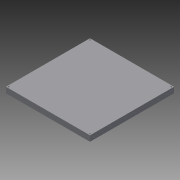
# Autodesk Inventor part: locomotion top
Saved by Autodesk Inventor 2015 (Build 190159000, 159)
## iProperties
Created: 2014-10-23
Part Number: locomotion top
Material: Generic
Document SubType Name: Modeling
Designer: ericd_000
Density: 1 g/cm^3
Appearance: Default
Author: ericd_000
Autodesk Inventor part; units mm, degrees
ref_plane "YZ Plane" through (0, 0, 0) normal (1, 0, 0) x (0, 1, 0)
ref_plane "XZ Plane" through (0, 0, 0) normal (0, 1, 0) x (-1, 0, 0)
ref_plane "XY Plane" through (0, 0, 0) normal (0, 0, 1) x (1, 0, 0)
sketch "Sketch1" plane through (0, 0, 0) normal (0, 0, 1) x (1, 0, 0)
  line L0 (-150, 150) -> (150, 150)
  line L1 (150, 150) -> (150, -150)
  line L2 (150, -150) -> (-150, -150)
  line L3 (-150, -150) -> (-150, 150)
  point P0 (0, 0)
  point P1 (0, 150)
  point P2 (150, 0)
  dimension "d0" = 300
  dimension "d1" = 300
  constraints: 8 end point, 2 midpoint, 2 parallel, 1 horizontal, 1 horizontal alignment, 1 perpendicular, 1 vertical alignment
  measures "d0" distance of L0.start L0.end
  measures "d1" distance of L2.end L0.start
extrude "Extrusion1" add sketch "Sketch1" along normal blind 10
sketch "Sketch2" plane through (0, 0, 0) normal (0, 0, -1) x (-1, 0, 0)
  line L0 (150, -150) -> (-150.0258, -150)
  line L1 (-150.0258, -150) -> (-150.0258, 150)
  line L2 (-150.0258, 150) -> (150, 150)
  line L3 (150, 150) -> (150, -150)
  line L4 (-140.0258, -140) -> (140, -140)
  line L5 (140, -140) -> (140, 140)
  line L6 (140, 140) -> (-140.0258, 140)
  line L7 (-140.0258, 140) -> (-140.0258, -140)
  point P0 (0, 0)
  dimension "d4" = 10
  constraints: 16 end point, 4 parallel, 2 perpendicular, 1 horizontal, 3 other
  measures "d4" distance between parallel lines of L3 L5
extrude "Extrusion2" add sketch "Sketch2" along normal blind 10
sketch "Sketch3" plane through (0, 0, 10) normal (0, 0, 1) x (1, 0, 0)
  circle A0 centre (-145, 145) radius 2.05
  circle A1 centre (145, 145) radius 2.05
  line L0 (-145, 145) -> (145, 145) construction
  line L1 (150, 150) -> (-150, 150) construction
  line L2 (-150, 150) -> (-150, -150) construction
  point P0 (0, 0)
  point P1 (0, 145)
  point P2 (0, 150)
  dimension "d7" = 5
  dimension "d8" = 4.1
  dimension "d9" = 4.1
  dimension "d10" = 5
  constraints: 2 centre point, 2 end point, 2 midpoint, 1 parallel, 1 vertical alignment
  measures "d7" distance from line of L2 L0.start
  measures "d8" diameter of A0
  measures "d9" diameter of A1
  measures "d10" distance between parallel lines of L1 L0
extrude "Extrusion3" cut sketch "Sketch3" against normal up to surface (20 mm away)
mirror "Mirror1" about plane through (0, 0, 0) normal (0, 1, 0) of "Extrusion3"
body "Solid1"
